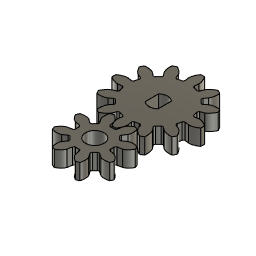
Assembly v13 (Autodesk Fusion 360 archive; units mm, degrees)
design "Gears"
description: Spur Gear; Module: 2.0; Num Teeth: 12; Pressure Angle: 20.0; Backlash: 0.00 mm
description: Spur Gear; Module: 2.000000; Num Teeth: 8; Pressure Angle: 20.000000; Backlash: 0.00 mm
Autodesk Fusion 360 part; units mm, degrees
(part 1 of 3)
sketch "Sketch1" plane through (0, 0.5, 0) normal (0, 0, -1) x (1, 0, 0)
  circle A0 centre (0, 0.5) radius 2.9
  arc A1 (11.3734, 7.8639) -> (11.1557, 8.1896) centre (0, 0.5) ccw
  arc A2 (11.3557, 9.5391) -> (11.1557, 8.1896) centre (11.9791, 8.7571) ccw
  line L0 (11.3557, 9.5391) -> (11.7631, 9.8639)
  spline S0 degree 5 poles (11.7631, 9.8639) (11.77, 9.8693) (11.7835, 9.8804) (11.8033, 9.8976) (11.8287, 9.9216) (11.8591, 9.953) (11.8887, 9.9854) (11.9177, 10.0186) (11.9463, 10.052) (11.9748, 10.0858) (12.003, 10.1198) (12.031, 10.1541) (12.0585, 10.1888) (12.0856, 10.2241) (12.1121, 10.2598) (12.1383, 10.296) (12.1641, 10.3326) (12.1895, 10.3695) (12.2147, 10.4067) (12.2396, 10.4442) (12.2642, 10.482) (12.2886, 10.52) (12.3126, 10.5583) (12.3363, 10.5969) (12.3598, 10.6358) (12.3829, 10.675) (12.4057, 10.7145) (12.4283, 10.7542) (12.4506, 10.7942) (12.4726, 10.8344) (12.4944, 10.8748) (12.5159, 10.9155) (12.5372, 10.9564) (12.5582, 10.9975) (12.5789, 11.0389) (12.5994, 11.0805) (12.6196, 11.1223) (12.6396, 11.1643) (12.6593, 11.2066) (12.6788, 11.249) (12.698, 11.2916) (12.717, 11.3345) (12.7358, 11.3775) (12.7543, 11.4207) (12.7725, 11.4642) (12.7905, 11.5078) (12.8083, 11.5516) (12.8259, 11.5955) (12.8432, 11.6397) (12.8603, 11.684) (12.8771, 11.7286) (12.8937, 11.7733) (12.9101, 11.8181) (12.9262, 11.8632) (12.9422, 11.9084) (12.9578, 11.9537) (12.9733, 11.9993) (12.9885, 12.045) (13.0035, 12.0908) (13.0183, 12.1368) (13.0328, 12.183) (13.0472, 12.2293) (13.0613, 12.2758) (13.0751, 12.3224) (13.0888, 12.3692) (13.1022, 12.4161) (13.1154, 12.4632) (13.1284, 12.5104) (13.1411, 12.5578) (13.1536, 12.6052) (13.1659, 12.6529) (13.1756, 12.6911) (13.1828, 12.7198) (13.1875, 12.739) (13.1898, 12.7486) knots 0 0 0 0 0 0 0.01428571 0.02857143 0.04285714 0.05714286 0.07142857 0.08571429 0.1 0.11428571 0.12857143 0.14285714 0.15714286 0.17142857 0.18571429 0.2 0.21428571 0.22857143 0.24285714 0.25714286 0.27142857 0.28571429 0.3 0.31428571 0.32857143 0.34285714 0.35714286 0.37142857 0.38571429 0.4 0.41428571 0.42857143 0.44285714 0.45714286 0.47142857 0.48571429 0.5 0.51428571 0.52857143 0.54285714 0.55714286 0.57142857 0.58571429 0.6 0.61428571 0.62857143 0.64285714 0.65714286 0.67142857 0.68571429 0.7 0.71428571 0.72857143 0.74285714 0.75714286 0.77142857 0.78571429 0.8 0.81428571 0.82857143 0.84285714 0.85714286 0.87142857 0.88571429 0.9 0.91428571 0.92857143 0.94285714 0.95714286 0.97142857 0.98571429 1 1 1 1 1 1
  arc A3 (13.1898, 12.7486) -> (12.2486, 13.6898) centre (0, 0.5) ccw
  spline S1 degree 5 poles (9.3639, 12.2631) (9.3693, 12.27) (9.3804, 12.2835) (9.3976, 12.3033) (9.4216, 12.3287) (9.453, 12.3591) (9.4854, 12.3887) (9.5186, 12.4177) (9.552, 12.4463) (9.5858, 12.4748) (9.6198, 12.503) (9.6541, 12.531) (9.6888, 12.5585) (9.7241, 12.5856) (9.7598, 12.6121) (9.796, 12.6383) (9.8326, 12.6641) (9.8695, 12.6895) (9.9067, 12.7147) (9.9442, 12.7396) (9.982, 12.7642) (10.02, 12.7886) (10.0583, 12.8126) (10.0969, 12.8363) (10.1358, 12.8598) (10.175, 12.8829) (10.2145, 12.9057) (10.2542, 12.9283) (10.2942, 12.9506) (10.3344, 12.9726) (10.3748, 12.9944) (10.4155, 13.0159) (10.4564, 13.0372) (10.4975, 13.0582) (10.5389, 13.0789) (10.5805, 13.0994) (10.6223, 13.1196) (10.6643, 13.1396) (10.7066, 13.1593) (10.749, 13.1788) (10.7916, 13.198) (10.8345, 13.217) (10.8775, 13.2358) (10.9207, 13.2543) (10.9642, 13.2725) (11.0078, 13.2905) (11.0516, 13.3083) (11.0955, 13.3259) (11.1397, 13.3432) (11.184, 13.3603) (11.2286, 13.3771) (11.2733, 13.3937) (11.3181, 13.4101) (11.3632, 13.4262) (11.4084, 13.4422) (11.4537, 13.4578) (11.4993, 13.4733) (11.545, 13.4885) (11.5908, 13.5035) (11.6368, 13.5183) (11.683, 13.5328) (11.7293, 13.5472) (11.7758, 13.5613) (11.8224, 13.5751) (11.8692, 13.5888) (11.9161, 13.6022) (11.9632, 13.6154) (12.0104, 13.6284) (12.0578, 13.6411) (12.1052, 13.6536) (12.1529, 13.6659) (12.1911, 13.6756) (12.2198, 13.6828) (12.239, 13.6875) (12.2486, 13.6898) knots 0 0 0 0 0 0 0.01428571 0.02857143 0.04285714 0.05714286 0.07142857 0.08571429 0.1 0.11428571 0.12857143 0.14285714 0.15714286 0.17142857 0.18571429 0.2 0.21428571 0.22857143 0.24285714 0.25714286 0.27142857 0.28571429 0.3 0.31428571 0.32857143 0.34285714 0.35714286 0.37142857 0.38571429 0.4 0.41428571 0.42857143 0.44285714 0.45714286 0.47142857 0.48571429 0.5 0.51428571 0.52857143 0.54285714 0.55714286 0.57142857 0.58571429 0.6 0.61428571 0.62857143 0.64285714 0.65714286 0.67142857 0.68571429 0.7 0.71428571 0.72857143 0.74285714 0.75714286 0.77142857 0.78571429 0.8 0.81428571 0.82857143 0.84285714 0.85714286 0.87142857 0.88571429 0.9 0.91428571 0.92857143 0.94285714 0.95714286 0.97142857 0.98571429 1 1 1 1 1 1
  line L1 (9.3639, 12.2631) -> (9.0391, 11.8557)
  arc A4 (7.6896, 11.6557) -> (9.0391, 11.8557) centre (8.2571, 12.4791) ccw
  arc A5 (7.6896, 11.6557) -> (7.3639, 11.8734) centre (0, 0.5) ccw
  arc A6 (7.0322, 13.1966) -> (7.3639, 11.8734) centre (7.9074, 12.7128) ccw
  line L2 (7.0322, 13.1966) -> (7.2843, 13.6527)
  spline S2 degree 5 poles (7.2843, 13.6527) (7.2886, 13.6603) (7.2968, 13.6757) (7.3085, 13.6992) (7.3228, 13.731) (7.3389, 13.7717) (7.3538, 13.813) (7.3679, 13.8547) (7.3816, 13.8966) (7.395, 13.9386) (7.408, 13.9808) (7.4207, 14.0232) (7.4328, 14.0659) (7.4444, 14.1088) (7.4552, 14.152) (7.4656, 14.1955) (7.4754, 14.2391) (7.4847, 14.283) (7.4938, 14.327) (7.5024, 14.3711) (7.5107, 14.4154) (7.5187, 14.4599) (7.5262, 14.5045) (7.5334, 14.5492) (7.5401, 14.5942) (7.5465, 14.6392) (7.5525, 14.6844) (7.5581, 14.7298) (7.5634, 14.7752) (7.5684, 14.8208) (7.573, 14.8665) (7.5774, 14.9123) (7.5813, 14.9582) (7.585, 15.0043) (7.5883, 15.0504) (7.5913, 15.0967) (7.594, 15.1431) (7.5964, 15.1895) (7.5984, 15.2361) (7.6002, 15.2827) (7.6017, 15.3295) (7.6028, 15.3763) (7.6037, 15.4233) (7.6042, 15.4703) (7.6045, 15.5174) (7.6044, 15.5646) (7.6041, 15.6118) (7.6035, 15.6592) (7.6026, 15.7066) (7.6014, 15.7541) (7.5999, 15.8017) (7.5982, 15.8493) (7.5961, 15.8971) (7.5938, 15.9448) (7.5912, 15.9927) (7.5883, 16.0406) (7.5852, 16.0886) (7.5818, 16.1366) (7.5781, 16.1847) (7.5741, 16.2329) (7.5699, 16.2811) (7.5654, 16.3294) (7.5606, 16.3777) (7.5556, 16.4261) (7.5503, 16.4746) (7.5447, 16.523) (7.5389, 16.5716) (7.5328, 16.6202) (7.5265, 16.6688) (7.5199, 16.7175) (7.513, 16.7662) (7.5073, 16.8052) (7.503, 16.8345) (7.5, 16.854) (7.4985, 16.8638) knots 0 0 0 0 0 0 0.01428571 0.02857143 0.04285714 0.05714286 0.07142857 0.08571429 0.1 0.11428571 0.12857143 0.14285714 0.15714286 0.17142857 0.18571429 0.2 0.21428571 0.22857143 0.24285714 0.25714286 0.27142857 0.28571429 0.3 0.31428571 0.32857143 0.34285714 0.35714286 0.37142857 0.38571429 0.4 0.41428571 0.42857143 0.44285714 0.45714286 0.47142857 0.48571429 0.5 0.51428571 0.52857143 0.54285714 0.55714286 0.57142857 0.58571429 0.6 0.61428571 0.62857143 0.64285714 0.65714286 0.67142857 0.68571429 0.7 0.71428571 0.72857143 0.74285714 0.75714286 0.77142857 0.78571429 0.8 0.81428571 0.82857143 0.84285714 0.85714286 0.87142857 0.88571429 0.9 0.91428571 0.92857143 0.94285714 0.95714286 0.97142857 0.98571429 1 1 1 1 1 1
  arc A7 (7.4985, 16.8638) -> (6.2687, 17.3732) centre (0, 0.5) ccw
  spline S3 degree 5 poles (4.1495, 14.9511) (4.152, 14.9595) (4.157, 14.9763) (4.1653, 15.0011) (4.1778, 15.0337) (4.1951, 15.0739) (4.2138, 15.1136) (4.2333, 15.1531) (4.2533, 15.1924) (4.2735, 15.2316) (4.2941, 15.2707) (4.3151, 15.3096) (4.3367, 15.3483) (4.3589, 15.3868) (4.3818, 15.4251) (4.4052, 15.4631) (4.4292, 15.5009) (4.4535, 15.5385) (4.4783, 15.576) (4.5034, 15.6134) (4.5288, 15.6506) (4.5546, 15.6876) (4.5808, 15.7245) (4.6074, 15.7612) (4.6344, 15.7977) (4.6618, 15.8341) (4.6895, 15.8703) (4.7176, 15.9064) (4.746, 15.9423) (4.7747, 15.978) (4.8037, 16.0136) (4.833, 16.049) (4.8627, 16.0843) (4.8927, 16.1195) (4.9229, 16.1545) (4.9535, 16.1893) (4.9844, 16.224) (5.0156, 16.2585) (5.0471, 16.2929) (5.0788, 16.3271) (5.1108, 16.3612) (5.1432, 16.3952) (5.1757, 16.4289) (5.2086, 16.4626) (5.2417, 16.4961) (5.2751, 16.5294) (5.3088, 16.5626) (5.3427, 16.5956) (5.3769, 16.6285) (5.4113, 16.6613) (5.446, 16.6939) (5.4809, 16.7263) (5.5161, 16.7586) (5.5515, 16.7908) (5.5872, 16.8228) (5.6231, 16.8546) (5.6593, 16.8863) (5.6957, 16.9179) (5.7323, 16.9493) (5.7691, 16.9806) (5.8062, 17.0117) (5.8435, 17.0426) (5.8811, 17.0734) (5.9189, 17.1041) (5.9569, 17.1346) (5.9951, 17.1649) (6.0335, 17.1951) (6.0722, 17.2252) (6.111, 17.2551) (6.1501, 17.2849) (6.1894, 17.3144) (6.221, 17.338) (6.2448, 17.3556) (6.2607, 17.3673) (6.2687, 17.3732) knots 0 0 0 0 0 0 0.01428571 0.02857143 0.04285714 0.05714286 0.07142857 0.08571429 0.1 0.11428571 0.12857143 0.14285714 0.15714286 0.17142857 0.18571429 0.2 0.21428571 0.22857143 0.24285714 0.25714286 0.27142857 0.28571429 0.3 0.31428571 0.32857143 0.34285714 0.35714286 0.37142857 0.38571429 0.4 0.41428571 0.42857143 0.44285714 0.45714286 0.47142857 0.48571429 0.5 0.51428571 0.52857143 0.54285714 0.55714286 0.57142857 0.58571429 0.6 0.61428571 0.62857143 0.64285714 0.65714286 0.67142857 0.68571429 0.7 0.71428571 0.72857143 0.74285714 0.75714286 0.77142857 0.78571429 0.8 0.81428571 0.82857143 0.84285714 0.85714286 0.87142857 0.88571429 0.9 0.91428571 0.92857143 0.94285714 0.95714286 0.97142857 0.98571429 1 1 1 1 1 1
  line L3 (4.1495, 14.9511) -> (4.0054, 14.4504)
  arc A8 (2.8352, 13.7493) -> (4.0054, 14.4504) centre (3.0444, 14.7271) ccw
  arc A9 (2.8352, 13.7493) -> (2.4509, 13.8257) centre (0, 0.5) ccw
  arc A10 (1.6381, 14.9213) -> (2.4509, 13.8257) centre (2.6318, 14.8092) ccw
  line L4 (1.6381, 14.9213) -> (1.6965, 15.4391)
  spline S4 degree 5 poles (1.6965, 15.4391) (1.6975, 15.4477) (1.6992, 15.4651) (1.7011, 15.4913) (1.7021, 15.5262) (1.7014, 15.57) (1.6994, 15.6138) (1.6964, 15.6577) (1.693, 15.7016) (1.6893, 15.7456) (1.6852, 15.7896) (1.6807, 15.8336) (1.6756, 15.8777) (1.6698, 15.9217) (1.6634, 15.9658) (1.6562, 16.0099) (1.6486, 16.054) (1.6405, 16.0981) (1.632, 16.1422) (1.6231, 16.1863) (1.6138, 16.2304) (1.6041, 16.2745) (1.594, 16.3186) (1.5835, 16.3627) (1.5726, 16.4068) (1.5612, 16.4508) (1.5494, 16.4949) (1.5373, 16.539) (1.5248, 16.583) (1.512, 16.627) (1.4988, 16.671) (1.4852, 16.715) (1.4713, 16.7589) (1.4571, 16.8029) (1.4425, 16.8468) (1.4276, 16.8907) (1.4123, 16.9345) (1.3967, 16.9784) (1.3808, 17.0222) (1.3646, 17.0659) (1.348, 17.1097) (1.3312, 17.1534) (1.314, 17.1971) (1.2965, 17.2407) (1.2787, 17.2844) (1.2606, 17.3279) (1.2422, 17.3715) (1.2235, 17.415) (1.2045, 17.4585) (1.1853, 17.5019) (1.1657, 17.5453) (1.1458, 17.5886) (1.1257, 17.6319) (1.1053, 17.6752) (1.0846, 17.7184) (1.0636, 17.7616) (1.0423, 17.8047) (1.0208, 17.8478) (0.9989, 17.8908) (0.9769, 17.9338) (0.9545, 17.9767) (0.9319, 18.0196) (0.909, 18.0624) (0.8858, 18.1052) (0.8624, 18.1479) (0.8387, 18.1906) (0.8147, 18.2332) (0.7905, 18.2758) (0.766, 18.3183) (0.7413, 18.3607) (0.7163, 18.4031) (0.6962, 18.437) (0.6809, 18.4623) (0.6707, 18.4792) (0.6655, 18.4877) knots 0 0 0 0 0 0 0.01428571 0.02857143 0.04285714 0.05714286 0.07142857 0.08571429 0.1 0.11428571 0.12857143 0.14285714 0.15714286 0.17142857 0.18571429 0.2 0.21428571 0.22857143 0.24285714 0.25714286 0.27142857 0.28571429 0.3 0.31428571 0.32857143 0.34285714 0.35714286 0.37142857 0.38571429 0.4 0.41428571 0.42857143 0.44285714 0.45714286 0.47142857 0.48571429 0.5 0.51428571 0.52857143 0.54285714 0.55714286 0.57142857 0.58571429 0.6 0.61428571 0.62857143 0.64285714 0.65714286 0.67142857 0.68571429 0.7 0.71428571 0.72857143 0.74285714 0.75714286 0.77142857 0.78571429 0.8 0.81428571 0.82857143 0.84285714 0.85714286 0.87142857 0.88571429 0.9 0.91428571 0.92857143 0.94285714 0.95714286 0.97142857 0.98571429 1 1 1 1 1 1
  arc A11 (0.6655, 18.4877) -> (-0.6655, 18.4877) centre (0, 0.5) ccw
  spline S5 degree 5 poles (-1.6965, 15.4391) (-1.6975, 15.4477) (-1.6992, 15.4651) (-1.7011, 15.4913) (-1.7021, 15.5262) (-1.7014, 15.57) (-1.6994, 15.6138) (-1.6964, 15.6577) (-1.693, 15.7016) (-1.6893, 15.7456) (-1.6852, 15.7896) (-1.6807, 15.8336) (-1.6756, 15.8777) (-1.6698, 15.9217) (-1.6634, 15.9658) (-1.6562, 16.0099) (-1.6486, 16.054) (-1.6405, 16.0981) (-1.632, 16.1422) (-1.6231, 16.1863) (-1.6138, 16.2304) (-1.6041, 16.2745) (-1.594, 16.3186) (-1.5835, 16.3627) (-1.5726, 16.4068) (-1.5612, 16.4508) (-1.5494, 16.4949) (-1.5373, 16.539) (-1.5248, 16.583) (-1.512, 16.627) (-1.4988, 16.671) (-1.4852, 16.715) (-1.4713, 16.7589) (-1.4571, 16.8029) (-1.4425, 16.8468) (-1.4276, 16.8907) (-1.4123, 16.9345) (-1.3967, 16.9784) (-1.3808, 17.0222) (-1.3646, 17.0659) (-1.348, 17.1097) (-1.3312, 17.1534) (-1.314, 17.1971) (-1.2965, 17.2407) (-1.2787, 17.2844) (-1.2606, 17.3279) (-1.2422, 17.3715) (-1.2235, 17.415) (-1.2045, 17.4585) (-1.1853, 17.5019) (-1.1657, 17.5453) (-1.1458, 17.5886) (-1.1257, 17.6319) (-1.1053, 17.6752) (-1.0846, 17.7184) (-1.0636, 17.7616) (-1.0423, 17.8047) (-1.0208, 17.8478) (-0.9989, 17.8908) (-0.9769, 17.9338) (-0.9545, 17.9767) (-0.9319, 18.0196) (-0.909, 18.0624) (-0.8858, 18.1052) (-0.8624, 18.1479) (-0.8387, 18.1906) (-0.8147, 18.2332) (-0.7905, 18.2758) (-0.766, 18.3183) (-0.7413, 18.3607) (-0.7163, 18.4031) (-0.6962, 18.437) (-0.6809, 18.4623) (-0.6707, 18.4792) (-0.6655, 18.4877) knots 0 0 0 0 0 0 0.01428571 0.02857143 0.04285714 0.05714286 0.07142857 0.08571429 0.1 0.11428571 0.12857143 0.14285714 0.15714286 0.17142857 0.18571429 0.2 0.21428571 0.22857143 0.24285714 0.25714286 0.27142857 0.28571429 0.3 0.31428571 0.32857143 0.34285714 0.35714286 0.37142857 0.38571429 0.4 0.41428571 0.42857143 0.44285714 0.45714286 0.47142857 0.48571429 0.5 0.51428571 0.52857143 0.54285714 0.55714286 0.57142857 0.58571429 0.6 0.61428571 0.62857143 0.64285714 0.65714286 0.67142857 0.68571429 0.7 0.71428571 0.72857143 0.74285714 0.75714286 0.77142857 0.78571429 0.8 0.81428571 0.82857143 0.84285714 0.85714286 0.87142857 0.88571429 0.9 0.91428571 0.92857143 0.94285714 0.95714286 0.97142857 0.98571429 1 1 1 1 1 1
  line L5 (-1.6965, 15.4391) -> (-1.6381, 14.9213)
  arc A12 (-2.4509, 13.8257) -> (-1.6381, 14.9213) centre (-2.6318, 14.8092) ccw
  arc A13 (-2.4509, 13.8257) -> (-2.8352, 13.7493) centre (0, 0.5) ccw
  arc A14 (-4.0054, 14.4504) -> (-2.8352, 13.7493) centre (-3.0444, 14.7271) ccw
  line L6 (-4.0054, 14.4504) -> (-4.1495, 14.9511)
  spline S6 degree 5 poles (-4.1495, 14.9511) (-4.152, 14.9595) (-4.157, 14.9763) (-4.1653, 15.0011) (-4.1778, 15.0337) (-4.1951, 15.0739) (-4.2138, 15.1136) (-4.2333, 15.1531) (-4.2533, 15.1924) (-4.2735, 15.2316) (-4.2941, 15.2707) (-4.3151, 15.3096) (-4.3367, 15.3483) (-4.3589, 15.3868) (-4.3818, 15.4251) (-4.4052, 15.4631) (-4.4292, 15.5009) (-4.4535, 15.5385) (-4.4783, 15.576) (-4.5034, 15.6134) (-4.5288, 15.6506) (-4.5546, 15.6876) (-4.5808, 15.7245) (-4.6074, 15.7612) (-4.6344, 15.7977) (-4.6618, 15.8341) (-4.6895, 15.8703) (-4.7176, 15.9064) (-4.746, 15.9423) (-4.7747, 15.978) (-4.8037, 16.0136) (-4.833, 16.049) (-4.8627, 16.0843) (-4.8927, 16.1195) (-4.9229, 16.1545) (-4.9535, 16.1893) (-4.9844, 16.224) (-5.0156, 16.2585) (-5.0471, 16.2929) (-5.0788, 16.3271) (-5.1108, 16.3612) (-5.1432, 16.3952) (-5.1757, 16.4289) (-5.2086, 16.4626) (-5.2417, 16.4961) (-5.2751, 16.5294) (-5.3088, 16.5626) (-5.3427, 16.5956) (-5.3769, 16.6285) (-5.4113, 16.6613) (-5.446, 16.6939) (-5.4809, 16.7263) (-5.5161, 16.7586) (-5.5515, 16.7908) (-5.5872, 16.8228) (-5.6231, 16.8546) (-5.6593, 16.8863) (-5.6957, 16.9179) (-5.7323, 16.9493) (-5.7691, 16.9806) (-5.8062, 17.0117) (-5.8435, 17.0426) (-5.8811, 17.0734) (-5.9189, 17.1041) (-5.9569, 17.1346) (-5.9951, 17.1649) (-6.0335, 17.1951) (-6.0722, 17.2252) (-6.111, 17.2551) (-6.1501, 17.2849) (-6.1894, 17.3144) (-6.221, 17.338) (-6.2448, 17.3556) (-6.2607, 17.3673) (-6.2687, 17.3732) knots 0 0 0 0 0 0 0.01428571 0.02857143 0.04285714 0.05714286 0.07142857 0.08571429 0.1 0.11428571 0.12857143 0.14285714 0.15714286 0.17142857 0.18571429 0.2 0.21428571 0.22857143 0.24285714 0.25714286 0.27142857 0.28571429 0.3 0.31428571 0.32857143 0.34285714 0.35714286 0.37142857 0.38571429 0.4 0.41428571 0.42857143 0.44285714 0.45714286 0.47142857 0.48571429 0.5 0.51428571 0.52857143 0.54285714 0.55714286 0.57142857 0.58571429 0.6 0.61428571 0.62857143 0.64285714 0.65714286 0.67142857 0.68571429 0.7 0.71428571 0.72857143 0.74285714 0.75714286 0.77142857 0.78571429 0.8 0.81428571 0.82857143 0.84285714 0.85714286 0.87142857 0.88571429 0.9 0.91428571 0.92857143 0.94285714 0.95714286 0.97142857 0.98571429 1 1 1 1 1 1
  arc A15 (-6.2687, 17.3732) -> (-7.4985, 16.8638) centre (0, 0.5) ccw
  spline S7 degree 5 poles (-7.2843, 13.6527) (-7.2886, 13.6603) (-7.2968, 13.6757) (-7.3085, 13.6992) (-7.3228, 13.731) (-7.3389, 13.7717) (-7.3538, 13.813) (-7.3679, 13.8547) (-7.3816, 13.8966) (-7.395, 13.9386) (-7.408, 13.9808) (-7.4207, 14.0232) (-7.4328, 14.0659) (-7.4444, 14.1088) (-7.4552, 14.152) (-7.4656, 14.1955) (-7.4754, 14.2391) (-7.4847, 14.283) (-7.4938, 14.327) (-7.5024, 14.3711) (-7.5107, 14.4154) (-7.5187, 14.4599) (-7.5262, 14.5045) (-7.5334, 14.5492) (-7.5401, 14.5942) (-7.5465, 14.6392) (-7.5525, 14.6844) (-7.5581, 14.7298) (-7.5634, 14.7752) (-7.5684, 14.8208) (-7.573, 14.8665) (-7.5774, 14.9123) (-7.5813, 14.9582) (-7.585, 15.0043) (-7.5883, 15.0504) (-7.5913, 15.0967) (-7.594, 15.1431) (-7.5964, 15.1895) (-7.5984, 15.2361) (-7.6002, 15.2827) (-7.6017, 15.3295) (-7.6028, 15.3763) (-7.6037, 15.4233) (-7.6042, 15.4703) (-7.6045, 15.5174) (-7.6044, 15.5646) (-7.6041, 15.6118) (-7.6035, 15.6592) (-7.6026, 15.7066) (-7.6014, 15.7541) (-7.5999, 15.8017) (-7.5982, 15.8493) (-7.5961, 15.8971) (-7.5938, 15.9448) (-7.5912, 15.9927) (-7.5883, 16.0406) (-7.5852, 16.0886) (-7.5818, 16.1366) (-7.5781, 16.1847) (-7.5741, 16.2329) (-7.5699, 16.2811) (-7.5654, 16.3294) (-7.5606, 16.3777) (-7.5556, 16.4261) (-7.5503, 16.4746) (-7.5447, 16.523) (-7.5389, 16.5716) (-7.5328, 16.6202) (-7.5265, 16.6688) (-7.5199, 16.7175) (-7.513, 16.7662) (-7.5073, 16.8052) (-7.503, 16.8345) (-7.5, 16.854) (-7.4985, 16.8638) knots 0 0 0 0 0 0 0.01428571 0.02857143 0.04285714 0.05714286 0.07142857 0.08571429 0.1 0.11428571 0.12857143 0.14285714 0.15714286 0.17142857 0.18571429 0.2 0.21428571 0.22857143 0.24285714 0.25714286 0.27142857 0.28571429 0.3 0.31428571 0.32857143 0.34285714 0.35714286 0.37142857 0.38571429 0.4 0.41428571 0.42857143 0.44285714 0.45714286 0.47142857 0.48571429 0.5 0.51428571 0.52857143 0.54285714 0.55714286 0.57142857 0.58571429 0.6 0.61428571 0.62857143 0.64285714 0.65714286 0.67142857 0.68571429 0.7 0.71428571 0.72857143 0.74285714 0.75714286 0.77142857 0.78571429 0.8 0.81428571 0.82857143 0.84285714 0.85714286 0.87142857 0.88571429 0.9 0.91428571 0.92857143 0.94285714 0.95714286 0.97142857 0.98571429 1 1 1 1 1 1
  line L7 (-7.2843, 13.6527) -> (-7.0322, 13.1966)
  arc A16 (-7.3639, 11.8734) -> (-7.0322, 13.1966) centre (-7.9074, 12.7128) ccw
  arc A17 (-7.3639, 11.8734) -> (-7.6896, 11.6557) centre (0, 0.5) ccw
  arc A18 (-9.0391, 11.8557) -> (-7.6896, 11.6557) centre (-8.2571, 12.4791) ccw
  line L8 (-9.0391, 11.8557) -> (-9.3639, 12.2631)
  spline S8 degree 5 poles (-9.3639, 12.2631) (-9.3693, 12.27) (-9.3804, 12.2835) (-9.3976, 12.3033) (-9.4216, 12.3287) (-9.453, 12.3591) (-9.4854, 12.3887) (-9.5186, 12.4177) (-9.552, 12.4463) (-9.5858, 12.4748) (-9.6198, 12.503) (-9.6541, 12.531) (-9.6888, 12.5585) (-9.7241, 12.5856) (-9.7598, 12.6121) (-9.796, 12.6383) (-9.8326, 12.6641) (-9.8695, 12.6895) (-9.9067, 12.7147) (-9.9442, 12.7396) (-9.982, 12.7642) (-10.02, 12.7886) (-10.0583, 12.8126) (-10.0969, 12.8363) (-10.1358, 12.8598) (-10.175, 12.8829) (-10.2145, 12.9057) (-10.2542, 12.9283) (-10.2942, 12.9506) (-10.3344, 12.9726) (-10.3748, 12.9944) (-10.4155, 13.0159) (-10.4564, 13.0372) (-10.4975, 13.0582) (-10.5389, 13.0789) (-10.5805, 13.0994) (-10.6223, 13.1196) (-10.6643, 13.1396) (-10.7066, 13.1593) (-10.749, 13.1788) (-10.7916, 13.198) (-10.8345, 13.217) (-10.8775, 13.2358) (-10.9207, 13.2543) (-10.9642, 13.2725) (-11.0078, 13.2905) (-11.0516, 13.3083) (-11.0955, 13.3259) (-11.1397, 13.3432) (-11.184, 13.3603) (-11.2286, 13.3771) (-11.2733, 13.3937) (-11.3181, 13.4101) (-11.3632, 13.4262) (-11.4084, 13.4422) (-11.4537, 13.4578) (-11.4993, 13.4733) (-11.545, 13.4885) (-11.5908, 13.5035) (-11.6368, 13.5183) (-11.683, 13.5328) (-11.7293, 13.5472) (-11.7758, 13.5613) (-11.8224, 13.5751) (-11.8692, 13.5888) (-11.9161, 13.6022) (-11.9632, 13.6154) (-12.0104, 13.6284) (-12.0578, 13.6411) (-12.1052, 13.6536) (-12.1529, 13.6659) (-12.1911, 13.6756) (-12.2198, 13.6828) (-12.239, 13.6875) (-12.2486, 13.6898) knots 0 0 0 0 0 0 0.01428571 0.02857143 0.04285714 0.05714286 0.07142857 0.08571429 0.1 0.11428571 0.12857143 0.14285714 0.15714286 0.17142857 0.18571429 0.2 0.21428571 0.22857143 0.24285714 0.25714286 0.27142857 0.28571429 0.3 0.31428571 0.32857143 0.34285714 0.35714286 0.37142857 0.38571429 0.4 0.41428571 0.42857143 0.44285714 0.45714286 0.47142857 0.48571429 0.5 0.51428571 0.52857143 0.54285714 0.55714286 0.57142857 0.58571429 0.6 0.61428571 0.62857143 0.64285714 0.65714286 0.67142857 0.68571429 0.7 0.71428571 0.72857143 0.74285714 0.75714286 0.77142857 0.78571429 0.8 0.81428571 0.82857143 0.84285714 0.85714286 0.87142857 0.88571429 0.9 0.91428571 0.92857143 0.94285714 0.95714286 0.97142857 0.98571429 1 1 1 1 1 1
  arc A19 (-12.2486, 13.6898) -> (-13.1898, 12.7486) centre (0, 0.5) ccw
  spline S9 degree 5 poles (-11.7631, 9.8639) (-11.77, 9.8693) (-11.7835, 9.8804) (-11.8033, 9.8976) (-11.8287, 9.9216) (-11.8591, 9.953) (-11.8887, 9.9854) (-11.9177, 10.0186) (-11.9463, 10.052) (-11.9748, 10.0858) (-12.003, 10.1198) (-12.031, 10.1541) (-12.0585, 10.1888) (-12.0856, 10.2241) (-12.1121, 10.2598) (-12.1383, 10.296) (-12.1641, 10.3326) (-12.1895, 10.3695) (-12.2147, 10.4067) (-12.2396, 10.4442) (-12.2642, 10.482) (-12.2886, 10.52) (-12.3126, 10.5583) (-12.3363, 10.5969) (-12.3598, 10.6358) (-12.3829, 10.675) (-12.4057, 10.7145) (-12.4283, 10.7542) (-12.4506, 10.7942) (-12.4726, 10.8344) (-12.4944, 10.8748) (-12.5159, 10.9155) (-12.5372, 10.9564) (-12.5582, 10.9975) (-12.5789, 11.0389) (-12.5994, 11.0805) (-12.6196, 11.1223) (-12.6396, 11.1643) (-12.6593, 11.2066) (-12.6788, 11.249) (-12.698, 11.2916) (-12.717, 11.3345) (-12.7358, 11.3775) (-12.7543, 11.4207) (-12.7725, 11.4642) (-12.7905, 11.5078) (-12.8083, 11.5516) (-12.8259, 11.5955) (-12.8432, 11.6397) (-12.8603, 11.684) (-12.8771, 11.7286) (-12.8937, 11.7733) (-12.9101, 11.8181) (-12.9262, 11.8632) (-12.9422, 11.9084) (-12.9578, 11.9537) (-12.9733, 11.9993) (-12.9885, 12.045) (-13.0035, 12.0908) (-13.0183, 12.1368) (-13.0328, 12.183) (-13.0472, 12.2293) (-13.0613, 12.2758) (-13.0751, 12.3224) (-13.0888, 12.3692) (-13.1022, 12.4161) (-13.1154, 12.4632) (-13.1284, 12.5104) (-13.1411, 12.5578) (-13.1536, 12.6052) (-13.1659, 12.6529) (-13.1756, 12.6911) (-13.1828, 12.7198) (-13.1875, 12.739) (-13.1898, 12.7486) knots 0 0 0 0 0 0 0.01428571 0.02857143 0.04285714 0.05714286 0.07142857 0.08571429 0.1 0.11428571 0.12857143 0.14285714 0.15714286 0.17142857 0.18571429 0.2 0.21428571 0.22857143 0.24285714 0.25714286 0.27142857 0.28571429 0.3 0.31428571 0.32857143 0.34285714 0.35714286 0.37142857 0.38571429 0.4 0.41428571 0.42857143 0.44285714 0.45714286 0.47142857 0.48571429 0.5 0.51428571 0.52857143 0.54285714 0.55714286 0.57142857 0.58571429 0.6 0.61428571 0.62857143 0.64285714 0.65714286 0.67142857 0.68571429 0.7 0.71428571 0.72857143 0.74285714 0.75714286 0.77142857 0.78571429 0.8 0.81428571 0.82857143 0.84285714 0.85714286 0.87142857 0.88571429 0.9 0.91428571 0.92857143 0.94285714 0.95714286 0.97142857 0.98571429 1 1 1 1 1 1
  line L9 (-11.7631, 9.8639) -> (-11.3557, 9.5391)
  arc A20 (-11.1557, 8.1896) -> (-11.3557, 9.5391) centre (-11.9791, 8.7571) ccw
  arc A21 (-11.1557, 8.1896) -> (-11.3734, 7.8639) centre (0, 0.5) ccw
  arc A22 (-12.6966, 7.5322) -> (-11.3734, 7.8639) centre (-12.2128, 8.4074) ccw
  line L10 (-12.6966, 7.5322) -> (-13.1527, 7.7843)
  spline S10 degree 5 poles (-13.1527, 7.7843) (-13.1603, 7.7886) (-13.1757, 7.7968) (-13.1992, 7.8085) (-13.231, 7.8228) (-13.2717, 7.8389) (-13.313, 7.8538) (-13.3547, 7.8679) (-13.3966, 7.8816) (-13.4386, 7.895) (-13.4808, 7.908) (-13.5232, 7.9207) (-13.5659, 7.9328) (-13.6088, 7.9444) (-13.652, 7.9552) (-13.6955, 7.9656) (-13.7391, 7.9754) (-13.783, 7.9847) (-13.827, 7.9938) (-13.8711, 8.0024) (-13.9154, 8.0107) (-13.9599, 8.0187) (-14.0045, 8.0262) (-14.0492, 8.0334) (-14.0942, 8.0401) (-14.1392, 8.0465) (-14.1844, 8.0525) (-14.2298, 8.0581) (-14.2752, 8.0634) (-14.3208, 8.0684) (-14.3665, 8.073) (-14.4123, 8.0774) (-14.4582, 8.0813) (-14.5043, 8.085) (-14.5504, 8.0883) (-14.5967, 8.0913) (-14.6431, 8.094) (-14.6895, 8.0964) (-14.7361, 8.0984) (-14.7827, 8.1002) (-14.8295, 8.1017) (-14.8763, 8.1028) (-14.9233, 8.1037) (-14.9703, 8.1042) (-15.0174, 8.1045) (-15.0646, 8.1044) (-15.1118, 8.1041) (-15.1592, 8.1035) (-15.2066, 8.1026) (-15.2541, 8.1014) (-15.3017, 8.0999) (-15.3493, 8.0982) (-15.3971, 8.0961) (-15.4448, 8.0938) (-15.4927, 8.0912) (-15.5406, 8.0883) (-15.5886, 8.0852) (-15.6366, 8.0818) (-15.6847, 8.0781) (-15.7329, 8.0741) (-15.7811, 8.0699) (-15.8294, 8.0654) (-15.8777, 8.0606) (-15.9261, 8.0556) (-15.9746, 8.0503) (-16.023, 8.0447) (-16.0716, 8.0389) (-16.1202, 8.0328) (-16.1688, 8.0265) (-16.2175, 8.0199) (-16.2662, 8.013) (-16.3052, 8.0073) (-16.3345, 8.003) (-16.354, 8) (-16.3638, 7.9985) knots 0 0 0 0 0 0 0.01428571 0.02857143 0.04285714 0.05714286 0.07142857 0.08571429 0.1 0.11428571 0.12857143 0.14285714 0.15714286 0.17142857 0.18571429 0.2 0.21428571 0.22857143 0.24285714 0.25714286 0.27142857 0.28571429 0.3 0.31428571 0.32857143 0.34285714 0.35714286 0.37142857 0.38571429 0.4 0.41428571 0.42857143 0.44285714 0.45714286 0.47142857 0.48571429 0.5 0.51428571 0.52857143 0.54285714 0.55714286 0.57142857 0.58571429 0.6 0.61428571 0.62857143 0.64285714 0.65714286 0.67142857 0.68571429 0.7 0.71428571 0.72857143 0.74285714 0.75714286 0.77142857 0.78571429 0.8 0.81428571 0.82857143 0.84285714 0.85714286 0.87142857 0.88571429 0.9 0.91428571 0.92857143 0.94285714 0.95714286 0.97142857 0.98571429 1 1 1 1 1 1
  arc A23 (-16.3638, 7.9985) -> (-16.8732, 6.7687) centre (0, 0.5) ccw
  spline S11 degree 5 poles (-14.4511, 4.6495) (-14.4595, 4.652) (-14.4763, 4.657) (-14.5011, 4.6653) (-14.5337, 4.6778) (-14.5739, 4.6951) (-14.6136, 4.7138) (-14.6531, 4.7333) (-14.6924, 4.7533) (-14.7316, 4.7735) (-14.7707, 4.7941) (-14.8096, 4.8151) (-14.8483, 4.8367) (-14.8868, 4.8589) (-14.9251, 4.8818) (-14.9631, 4.9052) (-15.0009, 4.9292) (-15.0385, 4.9535) (-15.076, 4.9783) (-15.1134, 5.0034) (-15.1506, 5.0288) (-15.1876, 5.0546) (-15.2245, 5.0808) (-15.2612, 5.1074) (-15.2977, 5.1344) (-15.3341, 5.1618) (-15.3703, 5.1895) (-15.4064, 5.2176) (-15.4423, 5.246) (-15.478, 5.2747) (-15.5136, 5.3037) (-15.549, 5.333) (-15.5843, 5.3627) (-15.6195, 5.3927) (-15.6545, 5.4229) (-15.6893, 5.4535) (-15.724, 5.4844) (-15.7585, 5.5156) (-15.7929, 5.5471) (-15.8271, 5.5788) (-15.8612, 5.6108) (-15.8952, 5.6432) (-15.9289, 5.6757) (-15.9626, 5.7086) (-15.9961, 5.7417) (-16.0294, 5.7751) (-16.0626, 5.8088) (-16.0956, 5.8427) (-16.1285, 5.8769) (-16.1613, 5.9113) (-16.1939, 5.946) (-16.2263, 5.9809) (-16.2586, 6.0161) (-16.2908, 6.0515) (-16.3228, 6.0872) (-16.3546, 6.1231) (-16.3863, 6.1593) (-16.4179, 6.1957) (-16.4493, 6.2323) (-16.4806, 6.2691) (-16.5117, 6.3062) (-16.5426, 6.3435) (-16.5734, 6.3811) (-16.6041, 6.4189) (-16.6346, 6.4569) (-16.6649, 6.4951) (-16.6951, 6.5335) (-16.7252, 6.5722) (-16.7551, 6.611) (-16.7849, 6.6501) (-16.8144, 6.6894) (-16.838, 6.721) (-16.8556, 6.7448) (-16.8673, 6.7607) (-16.8732, 6.7687) knots 0 0 0 0 0 0 0.01428571 0.02857143 0.04285714 0.05714286 0.07142857 0.08571429 0.1 0.11428571 0.12857143 0.14285714 0.15714286 0.17142857 0.18571429 0.2 0.21428571 0.22857143 0.24285714 0.25714286 0.27142857 0.28571429 0.3 0.31428571 0.32857143 0.34285714 0.35714286 0.37142857 0.38571429 0.4 0.41428571 0.42857143 0.44285714 0.45714286 0.47142857 0.48571429 0.5 0.51428571 0.52857143 0.54285714 0.55714286 0.57142857 0.58571429 0.6 0.61428571 0.62857143 0.64285714 0.65714286 0.67142857 0.68571429 0.7 0.71428571 0.72857143 0.74285714 0.75714286 0.77142857 0.78571429 0.8 0.81428571 0.82857143 0.84285714 0.85714286 0.87142857 0.88571429 0.9 0.91428571 0.92857143 0.94285714 0.95714286 0.97142857 0.98571429 1 1 1 1 1 1
  line L11 (-14.4511, 4.6495) -> (-13.9504, 4.5054)
  arc A24 (-13.2493, 3.3352) -> (-13.9504, 4.5054) centre (-14.2271, 3.5444) ccw
  arc A25 (-13.2493, 3.3352) -> (-13.3257, 2.9509) centre (0, 0.5) ccw
  arc A26 (-14.4213, 2.1381) -> (-13.3257, 2.9509) centre (-14.3092, 3.1318) ccw
  line L12 (-14.4213, 2.1381) -> (-14.9391, 2.1965)
  spline S12 degree 5 poles (-14.9391, 2.1965) (-14.9477, 2.1975) (-14.9651, 2.1992) (-14.9913, 2.2011) (-15.0262, 2.2021) (-15.07, 2.2014) (-15.1138, 2.1994) (-15.1577, 2.1964) (-15.2016, 2.193) (-15.2456, 2.1893) (-15.2896, 2.1852) (-15.3336, 2.1807) (-15.3777, 2.1756) (-15.4217, 2.1698) (-15.4658, 2.1634) (-15.5099, 2.1562) (-15.554, 2.1486) (-15.5981, 2.1405) (-15.6422, 2.132) (-15.6863, 2.1231) (-15.7304, 2.1138) (-15.7745, 2.1041) (-15.8186, 2.094) (-15.8627, 2.0835) (-15.9068, 2.0726) (-15.9508, 2.0612) (-15.9949, 2.0494) (-16.039, 2.0373) (-16.083, 2.0248) (-16.127, 2.012) (-16.171, 1.9988) (-16.215, 1.9852) (-16.2589, 1.9713) (-16.3029, 1.9571) (-16.3468, 1.9425) (-16.3907, 1.9276) (-16.4345, 1.9123) (-16.4784, 1.8967) (-16.5222, 1.8808) (-16.5659, 1.8646) (-16.6097, 1.848) (-16.6534, 1.8312) (-16.6971, 1.814) (-16.7407, 1.7965) (-16.7844, 1.7787) (-16.8279, 1.7606) (-16.8715, 1.7422) (-16.915, 1.7235) (-16.9585, 1.7045) (-17.0019, 1.6853) (-17.0453, 1.6657) (-17.0886, 1.6458) (-17.1319, 1.6257) (-17.1752, 1.6053) (-17.2184, 1.5846) (-17.2616, 1.5636) (-17.3047, 1.5423) (-17.3478, 1.5208) (-17.3908, 1.4989) (-17.4338, 1.4769) (-17.4767, 1.4545) (-17.5196, 1.4319) (-17.5624, 1.409) (-17.6052, 1.3858) (-17.6479, 1.3624) (-17.6906, 1.3387) (-17.7332, 1.3147) (-17.7758, 1.2905) (-17.8183, 1.266) (-17.8607, 1.2413) (-17.9031, 1.2163) (-17.937, 1.1962) (-17.9623, 1.1809) (-17.9792, 1.1707) (-17.9877, 1.1655) knots 0 0 0 0 0 0 0.01428571 0.02857143 0.04285714 0.05714286 0.07142857 0.08571429 0.1 0.11428571 0.12857143 0.14285714 0.15714286 0.17142857 0.18571429 0.2 0.21428571 0.22857143 0.24285714 0.25714286 0.27142857 0.28571429 0.3 0.31428571 0.32857143 0.34285714 0.35714286 0.37142857 0.38571429 0.4 0.41428571 0.42857143 0.44285714 0.45714286 0.47142857 0.48571429 0.5 0.51428571 0.52857143 0.54285714 0.55714286 0.57142857 0.58571429 0.6 0.61428571 0.62857143 0.64285714 0.65714286 0.67142857 0.68571429 0.7 0.71428571 0.72857143 0.74285714 0.75714286 0.77142857 0.78571429 0.8 0.81428571 0.82857143 0.84285714 0.85714286 0.87142857 0.88571429 0.9 0.91428571 0.92857143 0.94285714 0.95714286 0.97142857 0.98571429 1 1 1 1 1 1
  arc A27 (-17.9877, 1.1655) -> (-17.9877, -0.1655) centre (0, 0.5) ccw
  spline S13 degree 5 poles (-14.9391, -1.1965) (-14.9477, -1.1975) (-14.9651, -1.1992) (-14.9913, -1.2011) (-15.0262, -1.2021) (-15.07, -1.2014) (-15.1138, -1.1994) (-15.1577, -1.1964) (-15.2016, -1.193) (-15.2456, -1.1893) (-15.2896, -1.1852) (-15.3336, -1.1807) (-15.3777, -1.1756) (-15.4217, -1.1698) (-15.4658, -1.1634) (-15.5099, -1.1562) (-15.554, -1.1486) (-15.5981, -1.1405) (-15.6422, -1.132) (-15.6863, -1.1231) (-15.7304, -1.1138) (-15.7745, -1.1041) (-15.8186, -1.094) (-15.8627, -1.0835) (-15.9068, -1.0726) (-15.9508, -1.0612) (-15.9949, -1.0494) (-16.039, -1.0373) (-16.083, -1.0248) (-16.127, -1.012) (-16.171, -0.9988) (-16.215, -0.9852) (-16.2589, -0.9713) (-16.3029, -0.9571) (-16.3468, -0.9425) (-16.3907, -0.9276) (-16.4345, -0.9123) (-16.4784, -0.8967) (-16.5222, -0.8808) (-16.5659, -0.8646) (-16.6097, -0.848) (-16.6534, -0.8312) (-16.6971, -0.814) (-16.7407, -0.7965) (-16.7844, -0.7787) (-16.8279, -0.7606) (-16.8715, -0.7422) (-16.915, -0.7235) (-16.9585, -0.7045) (-17.0019, -0.6853) (-17.0453, -0.6657) (-17.0886, -0.6458) (-17.1319, -0.6257) (-17.1752, -0.6053) (-17.2184, -0.5846) (-17.2616, -0.5636) (-17.3047, -0.5423) (-17.3478, -0.5208) (-17.3908, -0.4989) (-17.4338, -0.4769) (-17.4767, -0.4545) (-17.5196, -0.4319) (-17.5624, -0.409) (-17.6052, -0.3858) (-17.6479, -0.3624) (-17.6906, -0.3387) (-17.7332, -0.3147) (-17.7758, -0.2905) (-17.8183, -0.266) (-17.8607, -0.2413) (-17.9031, -0.2163) (-17.937, -0.1962) (-17.9623, -0.1809) (-17.9792, -0.1707) (-17.9877, -0.1655) knots 0 0 0 0 0 0 0.01428571 0.02857143 0.04285714 0.05714286 0.07142857 0.08571429 0.1 0.11428571 0.12857143 0.14285714 0.15714286 0.17142857 0.18571429 0.2 0.21428571 0.22857143 0.24285714 0.25714286 0.27142857 0.28571429 0.3 0.31428571 0.32857143 0.34285714 0.35714286 0.37142857 0.38571429 0.4 0.41428571 0.42857143 0.44285714 0.45714286 0.47142857 0.48571429 0.5 0.51428571 0.52857143 0.54285714 0.55714286 0.57142857 0.58571429 0.6 0.61428571 0.62857143 0.64285714 0.65714286 0.67142857 0.68571429 0.7 0.71428571 0.72857143 0.74285714 0.75714286 0.77142857 0.78571429 0.8 0.81428571 0.82857143 0.84285714 0.85714286 0.87142857 0.88571429 0.9 0.91428571 0.92857143 0.94285714 0.95714286 0.97142857 0.98571429 1 1 1 1 1 1
  line L13 (-14.9391, -1.1965) -> (-14.4213, -1.1381)
  arc A28 (-13.3257, -1.9509) -> (-14.4213, -1.1381) centre (-14.3092, -2.1318) ccw
  arc A29 (-13.3257, -1.9509) -> (-13.2493, -2.3352) centre (0, 0.5) ccw
  arc A30 (-13.9504, -3.5054) -> (-13.2493, -2.3352) centre (-14.2271, -2.5444) ccw
  line L14 (-13.9504, -3.5054) -> (-14.4511, -3.6495)
  spline S14 degree 5 poles (-14.4511, -3.6495) (-14.4595, -3.652) (-14.4763, -3.657) (-14.5011, -3.6653) (-14.5337, -3.6778) (-14.5739, -3.6951) (-14.6136, -3.7138) (-14.6531, -3.7333) (-14.6924, -3.7533) (-14.7316, -3.7735) (-14.7707, -3.7941) (-14.8096, -3.8151) (-14.8483, -3.8367) (-14.8868, -3.8589) (-14.9251, -3.8818) (-14.9631, -3.9052) (-15.0009, -3.9292) (-15.0385, -3.9535) (-15.076, -3.9783) (-15.1134, -4.0034) (-15.1506, -4.0288) (-15.1876, -4.0546) (-15.2245, -4.0808) (-15.2612, -4.1074) (-15.2977, -4.1344) (-15.3341, -4.1618) (-15.3703, -4.1895) (-15.4064, -4.2176) (-15.4423, -4.246) (-15.478, -4.2747) (-15.5136, -4.3037) (-15.549, -4.333) (-15.5843, -4.3627) (-15.6195, -4.3927) (-15.6545, -4.4229) (-15.6893, -4.4535) (-15.724, -4.4844) (-15.7585, -4.5156) (-15.7929, -4.5471) (-15.8271, -4.5788) (-15.8612, -4.6108) (-15.8952, -4.6432) (-15.9289, -4.6757) (-15.9626, -4.7086) (-15.9961, -4.7417) (-16.0294, -4.7751) (-16.0626, -4.8088) (-16.0956, -4.8427) (-16.1285, -4.8769) (-16.1613, -4.9113) (-16.1939, -4.946) (-16.2263, -4.9809) (-16.2586, -5.0161) (-16.2908, -5.0515) (-16.3228, -5.0872) (-16.3546, -5.1231) (-16.3863, -5.1593) (-16.4179, -5.1957) (-16.4493, -5.2323) (-16.4806, -5.2691) (-16.5117, -5.3062) (-16.5426, -5.3435) (-16.5734, -5.3811) (-16.6041, -5.4189) (-16.6346, -5.4569) (-16.6649, -5.4951) (-16.6951, -5.5335) (-16.7252, -5.5722) (-16.7551, -5.611) (-16.7849, -5.6501) (-16.8144, -5.6894) (-16.838, -5.721) (-16.8556, -5.7448) (-16.8673, -5.7607) (-16.8732, -5.7687) knots 0 0 0 0 0 0 0.01428571 0.02857143 0.04285714 0.05714286 0.07142857 0.08571429 0.1 0.11428571 0.12857143 0.14285714 0.15714286 0.17142857 0.18571429 0.2 0.21428571 0.22857143 0.24285714 0.25714286 0.27142857 0.28571429 0.3 0.31428571 0.32857143 0.34285714 0.35714286 0.37142857 0.38571429 0.4 0.41428571 0.42857143 0.44285714 0.45714286 0.47142857 0.48571429 0.5 0.51428571 0.52857143 0.54285714 0.55714286 0.57142857 0.58571429 0.6 0.61428571 0.62857143 0.64285714 0.65714286 0.67142857 0.68571429 0.7 0.71428571 0.72857143 0.74285714 0.75714286 0.77142857 0.78571429 0.8 0.81428571 0.82857143 0.84285714 0.85714286 0.87142857 0.88571429 0.9 0.91428571 0.92857143 0.94285714 0.95714286 0.97142857 0.98571429 1 1 1 1 1 1
  arc A31 (-16.8732, -5.7687) -> (-16.3638, -6.9985) centre (0, 0.5) ccw
  spline S15 degree 5 poles (-13.1527, -6.7843) (-13.1603, -6.7886) (-13.1757, -6.7968) (-13.1992, -6.8085) (-13.231, -6.8228) (-13.2717, -6.8389) (-13.313, -6.8538) (-13.3547, -6.8679) (-13.3966, -6.8816) (-13.4386, -6.895) (-13.4808, -6.908) (-13.5232, -6.9207) (-13.5659, -6.9328) (-13.6088, -6.9444) (-13.652, -6.9552) (-13.6955, -6.9656) (-13.7391, -6.9754) (-13.783, -6.9847) (-13.827, -6.9938) (-13.8711, -7.0024) (-13.9154, -7.0107) (-13.9599, -7.0187) (-14.0045, -7.0262) (-14.0492, -7.0334) (-14.0942, -7.0401) (-14.1392, -7.0465) (-14.1844, -7.0525) (-14.2298, -7.0581) (-14.2752, -7.0634) (-14.3208, -7.0684) (-14.3665, -7.073) (-14.4123, -7.0774) (-14.4582, -7.0813) (-14.5043, -7.085) (-14.5504, -7.0883) (-14.5967, -7.0913) (-14.6431, -7.094) (-14.6895, -7.0964) (-14.7361, -7.0984) (-14.7827, -7.1002) (-14.8295, -7.1017) (-14.8763, -7.1028) (-14.9233, -7.1037) (-14.9703, -7.1042) (-15.0174, -7.1045) (-15.0646, -7.1044) (-15.1118, -7.1041) (-15.1592, -7.1035) (-15.2066, -7.1026) (-15.2541, -7.1014) (-15.3017, -7.0999) (-15.3493, -7.0982) (-15.3971, -7.0961) (-15.4448, -7.0938) (-15.4927, -7.0912) (-15.5406, -7.0883) (-15.5886, -7.0852) (-15.6366, -7.0818) (-15.6847, -7.0781) (-15.7329, -7.0741) (-15.7811, -7.0699) (-15.8294, -7.0654) (-15.8777, -7.0606) (-15.9261, -7.0556) (-15.9746, -7.0503) (-16.023, -7.0447) (-16.0716, -7.0389) (-16.1202, -7.0328) (-16.1688, -7.0265) (-16.2175, -7.0199) (-16.2662, -7.013) (-16.3052, -7.0073) (-16.3345, -7.003) (-16.354, -7) (-16.3638, -6.9985) knots 0 0 0 0 0 0 0.01428571 0.02857143 0.04285714 0.05714286 0.07142857 0.08571429 0.1 0.11428571 0.12857143 0.14285714 0.15714286 0.17142857 0.18571429 0.2 0.21428571 0.22857143 0.24285714 0.25714286 0.27142857 0.28571429 0.3 0.31428571 0.32857143 0.34285714 0.35714286 0.37142857 0.38571429 0.4 0.41428571 0.42857143 0.44285714 0.45714286 0.47142857 0.48571429 0.5 0.51428571 0.52857143 0.54285714 0.55714286 0.57142857 0.58571429 0.6 0.61428571 0.62857143 0.64285714 0.65714286 0.67142857 0.68571429 0.7 0.71428571 0.72857143 0.74285714 0.75714286 0.77142857 0.78571429 0.8 0.81428571 0.82857143 0.84285714 0.85714286 0.87142857 0.88571429 0.9 0.91428571 0.92857143 0.94285714 0.95714286 0.97142857 0.98571429 1 1 1 1 1 1
  line L15 (-13.1527, -6.7843) -> (-12.6966, -6.5322)
  arc A32 (-11.3734, -6.8639) -> (-12.6966, -6.5322) centre (-12.2128, -7.4074) ccw
  arc A33 (-11.3734, -6.8639) -> (-11.1557, -7.1896) centre (0, 0.5) ccw
  arc A34 (-11.3557, -8.5391) -> (-11.1557, -7.1896) centre (-11.9791, -7.7571) ccw
  line L16 (-11.3557, -8.5391) -> (-11.7631, -8.8639)
  spline S16 degree 5 poles (-11.7631, -8.8639) (-11.77, -8.8693) (-11.7835, -8.8804) (-11.8033, -8.8976) (-11.8287, -8.9216) (-11.8591, -8.953) (-11.8887, -8.9854) (-11.9177, -9.0186) (-11.9463, -9.052) (-11.9748, -9.0858) (-12.003, -9.1198) (-12.031, -9.1541) (-12.0585, -9.1888) (-12.0856, -9.2241) (-12.1121, -9.2598) (-12.1383, -9.296) (-12.1641, -9.3326) (-12.1895, -9.3695) (-12.2147, -9.4067) (-12.2396, -9.4442) (-12.2642, -9.482) (-12.2886, -9.52) (-12.3126, -9.5583) (-12.3363, -9.5969) (-12.3598, -9.6358) (-12.3829, -9.675) (-12.4057, -9.7145) (-12.4283, -9.7542) (-12.4506, -9.7942) (-12.4726, -9.8344) (-12.4944, -9.8748) (-12.5159, -9.9155) (-12.5372, -9.9564) (-12.5582, -9.9975) (-12.5789, -10.0389) (-12.5994, -10.0805) (-12.6196, -10.1223) (-12.6396, -10.1643) (-12.6593, -10.2066) (-12.6788, -10.249) (-12.698, -10.2916) (-12.717, -10.3345) (-12.7358, -10.3775) (-12.7543, -10.4207) (-12.7725, -10.4642) (-12.7905, -10.5078) (-12.8083, -10.5516) (-12.8259, -10.5955) (-12.8432, -10.6397) (-12.8603, -10.684) (-12.8771, -10.7286) (-12.8937, -10.7733) (-12.9101, -10.8181) (-12.9262, -10.8632) (-12.9422, -10.9084) (-12.9578, -10.9537) (-12.9733, -10.9993) (-12.9885, -11.045) (-13.0035, -11.0908) (-13.0183, -11.1368) (-13.0328, -11.183) (-13.0472, -11.2293) (-13.0613, -11.2758) (-13.0751, -11.3224) (-13.0888, -11.3692) (-13.1022, -11.4161) (-13.1154, -11.4632) (-13.1284, -11.5104) (-13.1411, -11.5578) (-13.1536, -11.6052) (-13.1659, -11.6529) (-13.1756, -11.6911) (-13.1828, -11.7198) (-13.1875, -11.739) (-13.1898, -11.7486) knots 0 0 0 0 0 0 0.01428571 0.02857143 0.04285714 0.05714286 0.07142857 0.08571429 0.1 0.11428571 0.12857143 0.14285714 0.15714286 0.17142857 0.18571429 0.2 0.21428571 0.22857143 0.24285714 0.25714286 0.27142857 0.28571429 0.3 0.31428571 0.32857143 0.34285714 0.35714286 0.37142857 0.38571429 0.4 0.41428571 0.42857143 0.44285714 0.45714286 0.47142857 0.48571429 0.5 0.51428571 0.52857143 0.54285714 0.55714286 0.57142857 0.58571429 0.6 0.61428571 0.62857143 0.64285714 0.65714286 0.67142857 0.68571429 0.7 0.71428571 0.72857143 0.74285714 0.75714286 0.77142857 0.78571429 0.8 0.81428571 0.82857143 0.84285714 0.85714286 0.87142857 0.88571429 0.9 0.91428571 0.92857143 0.94285714 0.95714286 0.97142857 0.98571429 1 1 1 1 1 1
  arc A35 (-13.1898, -11.7486) -> (-12.2486, -12.6898) centre (0, 0.5) ccw
  spline S17 degree 5 poles (-9.3639, -11.2631) (-9.3693, -11.27) (-9.3804, -11.2835) (-9.3976, -11.3033) (-9.4216, -11.3287) (-9.453, -11.3591) (-9.4854, -11.3887) (-9.5186, -11.4177) (-9.552, -11.4463) (-9.5858, -11.4748) (-9.6198, -11.503) (-9.6541, -11.531) (-9.6888, -11.5585) (-9.7241, -11.5856) (-9.7598, -11.6121) (-9.796, -11.6383) (-9.8326, -11.6641) (-9.8695, -11.6895) (-9.9067, -11.7147) (-9.9442, -11.7396) (-9.982, -11.7642) (-10.02, -11.7886) (-10.0583, -11.8126) (-10.0969, -11.8363) (-10.1358, -11.8598) (-10.175, -11.8829) (-10.2145, -11.9057) (-10.2542, -11.9283) (-10.2942, -11.9506) (-10.3344, -11.9726) (-10.3748, -11.9944) (-10.4155, -12.0159) (-10.4564, -12.0372) (-10.4975, -12.0582) (-10.5389, -12.0789) (-10.5805, -12.0994) (-10.6223, -12.1196) (-10.6643, -12.1396) (-10.7066, -12.1593) (-10.749, -12.1788) (-10.7916, -12.198) (-10.8345, -12.217) (-10.8775, -12.2358) (-10.9207, -12.2543) (-10.9642, -12.2725) (-11.0078, -12.2905) (-11.0516, -12.3083) (-11.0955, -12.3259) (-11.1397, -12.3432) (-11.184, -12.3603) (-11.2286, -12.3771) (-11.2733, -12.3937) (-11.3181, -12.4101) (-11.3632, -12.4262) (-11.4084, -12.4422) (-11.4537, -12.4578) (-11.4993, -12.4733) (-11.545, -12.4885) (-11.5908, -12.5035) (-11.6368, -12.5183) (-11.683, -12.5328) (-11.7293, -12.5472) (-11.7758, -12.5613) (-11.8224, -12.5751) (-11.8692, -12.5888) (-11.9161, -12.6022) (-11.9632, -12.6154) (-12.0104, -12.6284) (-12.0578, -12.6411) (-12.1052, -12.6536) (-12.1529, -12.6659) (-12.1911, -12.6756) (-12.2198, -12.6828) (-12.239, -12.6875) (-12.2486, -12.6898) knots 0 0 0 0 0 0 0.01428571 0.02857143 0.04285714 0.05714286 0.07142857 0.08571429 0.1 0.11428571 0.12857143 0.14285714 0.15714286 0.17142857 0.18571429 0.2 0.21428571 0.22857143 0.24285714 0.25714286 0.27142857 0.28571429 0.3 0.31428571 0.32857143 0.34285714 0.35714286 0.37142857 0.38571429 0.4 0.41428571 0.42857143 0.44285714 0.45714286 0.47142857 0.48571429 0.5 0.51428571 0.52857143 0.54285714 0.55714286 0.57142857 0.58571429 0.6 0.61428571 0.62857143 0.64285714 0.65714286 0.67142857 0.68571429 0.7 0.71428571 0.72857143 0.74285714 0.75714286 0.77142857 0.78571429 0.8 0.81428571 0.82857143 0.84285714 0.85714286 0.87142857 0.88571429 0.9 0.91428571 0.92857143 0.94285714 0.95714286 0.97142857 0.98571429 1 1 1 1 1 1
  line L17 (-9.3639, -11.2631) -> (-9.0391, -10.8557)
  arc A36 (-7.6896, -10.6557) -> (-9.0391, -10.8557) centre (-8.2571, -11.4791) ccw
  arc A37 (-7.6896, -10.6557) -> (-7.3639, -10.8734) centre (0, 0.5) ccw
  arc A38 (-7.0322, -12.1966) -> (-7.3639, -10.8734) centre (-7.9074, -11.7128) ccw
  line L18 (-7.0322, -12.1966) -> (-7.2843, -12.6527)
  spline S18 degree 5 poles (-7.2843, -12.6527) (-7.2886, -12.6603) (-7.2968, -12.6757) (-7.3085, -12.6992) (-7.3228, -12.731) (-7.3389, -12.7717) (-7.3538, -12.813) (-7.3679, -12.8547) (-7.3816, -12.8966) (-7.395, -12.9386) (-7.408, -12.9808) (-7.4207, -13.0232) (-7.4328, -13.0659) (-7.4444, -13.1088) (-7.4552, -13.152) (-7.4656, -13.1955) (-7.4754, -13.2391) (-7.4847, -13.283) (-7.4938, -13.327) (-7.5024, -13.3711) (-7.5107, -13.4154) (-7.5187, -13.4599) (-7.5262, -13.5045) (-7.5334, -13.5492) (-7.5401, -13.5942) (-7.5465, -13.6392) (-7.5525, -13.6844) (-7.5581, -13.7298) (-7.5634, -13.7752) (-7.5684, -13.8208) (-7.573, -13.8665) (-7.5774, -13.9123) (-7.5813, -13.9582) (-7.585, -14.0043) (-7.5883, -14.0504) (-7.5913, -14.0967) (-7.594, -14.1431) (-7.5964, -14.1895) (-7.5984, -14.2361) (-7.6002, -14.2827) (-7.6017, -14.3295) (-7.6028, -14.3763) (-7.6037, -14.4233) (-7.6042, -14.4703) (-7.6045, -14.5174) (-7.6044, -14.5646) (-7.6041, -14.6118) (-7.6035, -14.6592) (-7.6026, -14.7066) (-7.6014, -14.7541) (-7.5999, -14.8017) (-7.5982, -14.8493) (-7.5961, -14.8971) (-7.5938, -14.9448) (-7.5912, -14.9927) (-7.5883, -15.0406) (-7.5852, -15.0886) (-7.5818, -15.1366) (-7.5781, -15.1847) (-7.5741, -15.2329) (-7.5699, -15.2811) (-7.5654, -15.3294) (-7.5606, -15.3777) (-7.5556, -15.4261) (-7.5503, -15.4746) (-7.5447, -15.523) (-7.5389, -15.5716) (-7.5328, -15.6202) (-7.5265, -15.6688) (-7.5199, -15.7175) (-7.513, -15.7662) (-7.5073, -15.8052) (-7.503, -15.8345) (-7.5, -15.854) (-7.4985, -15.8638) knots 0 0 0 0 0 0 0.01428571 0.02857143 0.04285714 0.05714286 0.07142857 0.08571429 0.1 0.11428571 0.12857143 0.14285714 0.15714286 0.17142857 0.18571429 0.2 0.21428571 0.22857143 0.24285714 0.25714286 0.27142857 0.28571429 0.3 0.31428571 0.32857143 0.34285714 0.35714286 0.37142857 0.38571429 0.4 0.41428571 0.42857143 0.44285714 0.45714286 0.47142857 0.48571429 0.5 0.51428571 0.52857143 0.54285714 0.55714286 0.57142857 0.58571429 0.6 0.61428571 0.62857143 0.64285714 0.65714286 0.67142857 0.68571429 0.7 0.71428571 0.72857143 0.74285714 0.75714286 0.77142857 0.78571429 0.8 0.81428571 0.82857143 0.84285714 0.85714286 0.87142857 0.88571429 0.9 0.91428571 0.92857143 0.94285714 0.95714286 0.97142857 0.98571429 1 1 1 1 1 1
  arc A39 (-7.4985, -15.8638) -> (-6.2687, -16.3732) centre (0, 0.5) ccw
  spline S19 degree 5 poles (-4.1495, -13.9511) (-4.152, -13.9595) (-4.157, -13.9763) (-4.1653, -14.0011) (-4.1778, -14.0337) (-4.1951, -14.0739) (-4.2138, -14.1136) (-4.2333, -14.1531) (-4.2533, -14.1924) (-4.2735, -14.2316) (-4.2941, -14.2707) (-4.3151, -14.3096) (-4.3367, -14.3483) (-4.3589, -14.3868) (-4.3818, -14.4251) (-4.4052, -14.4631) (-4.4292, -14.5009) (-4.4535, -14.5385) (-4.4783, -14.576) (-4.5034, -14.6134) (-4.5288, -14.6506) (-4.5546, -14.6876) (-4.5808, -14.7245) (-4.6074, -14.7612) (-4.6344, -14.7977) (-4.6618, -14.8341) (-4.6895, -14.8703) (-4.7176, -14.9064) (-4.746, -14.9423) (-4.7747, -14.978) (-4.8037, -15.0136) (-4.833, -15.049) (-4.8627, -15.0843) (-4.8927, -15.1195) (-4.9229, -15.1545) (-4.9535, -15.1893) (-4.9844, -15.224) (-5.0156, -15.2585) (-5.0471, -15.2929) (-5.0788, -15.3271) (-5.1108, -15.3612) (-5.1432, -15.3952) (-5.1757, -15.4289) (-5.2086, -15.4626) (-5.2417, -15.4961) (-5.2751, -15.5294) (-5.3088, -15.5626) (-5.3427, -15.5956) (-5.3769, -15.6285) (-5.4113, -15.6613) (-5.446, -15.6939) (-5.4809, -15.7263) (-5.5161, -15.7586) (-5.5515, -15.7908) (-5.5872, -15.8228) (-5.6231, -15.8546) (-5.6593, -15.8863) (-5.6957, -15.9179) (-5.7323, -15.9493) (-5.7691, -15.9806) (-5.8062, -16.0117) (-5.8435, -16.0426) (-5.8811, -16.0734) (-5.9189, -16.1041) (-5.9569, -16.1346) (-5.9951, -16.1649) (-6.0335, -16.1951) (-6.0722, -16.2252) (-6.111, -16.2551) (-6.1501, -16.2849) (-6.1894, -16.3144) (-6.221, -16.338) (-6.2448, -16.3556) (-6.2607, -16.3673) (-6.2687, -16.3732) knots 0 0 0 0 0 0 0.01428571 0.02857143 0.04285714 0.05714286 0.07142857 0.08571429 0.1 0.11428571 0.12857143 0.14285714 0.15714286 0.17142857 0.18571429 0.2 0.21428571 0.22857143 0.24285714 0.25714286 0.27142857 0.28571429 0.3 0.31428571 0.32857143 0.34285714 0.35714286 0.37142857 0.38571429 0.4 0.41428571 0.42857143 0.44285714 0.45714286 0.47142857 0.48571429 0.5 0.51428571 0.52857143 0.54285714 0.55714286 0.57142857 0.58571429 0.6 0.61428571 0.62857143 0.64285714 0.65714286 0.67142857 0.68571429 0.7 0.71428571 0.72857143 0.74285714 0.75714286 0.77142857 0.78571429 0.8 0.81428571 0.82857143 0.84285714 0.85714286 0.87142857 0.88571429 0.9 0.91428571 0.92857143 0.94285714 0.95714286 0.97142857 0.98571429 1 1 1 1 1 1
  line L19 (-4.1495, -13.9511) -> (-4.0054, -13.4504)
  arc A40 (-2.8352, -12.7493) -> (-4.0054, -13.4504) centre (-3.0444, -13.7271) ccw
  arc A41 (-2.8352, -12.7493) -> (-2.4509, -12.8257) centre (0, 0.5) ccw
  arc A42 (-1.6381, -13.9213) -> (-2.4509, -12.8257) centre (-2.6318, -13.8092) ccw
  line L20 (-1.6381, -13.9213) -> (-1.6965, -14.4391)